Autodesk Fusion 360 part; units mm, degrees
(part 2 of 2)
sketch "Sketch1" plane through (0, 0, 0) normal (0, 0, 1) x (1, 0, 0)
  circle A0 centre (0, 0) radius 13.65
  circle A1 centre (0, 0) radius 18.65
  line L0 (0, 0) -> (0, 18.65)
  line L1 (0, 0) -> (0, -18.65)
  line L2 (-0.5, -18.6433) -> (-0.5, 18.6433)
  line L3 (-0.5, 18.6433) -> (-0.5, 25.4071)
  line L4 (-0.5, 25.4071) -> (-3, 25.4071)
  line L5 (-3, 25.4071) -> (-3, 18.4071)
  line L6 (0, 0) -> (-1.65, 0) construction
  line L7 (-1.65, 0) -> (-18.65, 0) construction
  line L8 (-18.216, 4) -> (-32, 4)
  line L9 (-32, 4) -> (-32, -4)
  line L10 (-32, -4) -> (-18.216, -4)
  circle A2 centre (-28, 0) radius 2.5
  circle A3 centre (-22, 0) radius 2.5
  line L11 (-22, -2.5) -> (-28, -2.5)
  line L12 (-28, 2.5) -> (-22, 2.5)
  line L13 (0.5, -18.6433) -> (0.5, 18.6433)
  line L14 (0.5, 18.6433) -> (0.5, 25.4071)
  line L15 (0.5, 25.4071) -> (3, 25.4071)
  line L16 (3, 25.4071) -> (3, 18.4071)
  line L17 (18.216, 4) -> (32, 4)
  circle A4 centre (22, 0) radius 2.5
  line L18 (28, 2.5) -> (22, 2.5)
  line L19 (22, -2.5) -> (28, -2.5)
  circle A5 centre (28, 0) radius 2.5
  line L20 (32, -4) -> (18.216, -4)
  line L21 (32, 4) -> (32, -4)
  dimension "d1" = 27.3
  dimension "d2" = 5
  dimension "d3" = 0.5
  dimension "d4" = 2.5
  dimension "d5" = 7
  dimension "d6" = 8
  dimension "d7" = 4
  dimension "d8" = 32
  dimension "d9" = 5
  dimension "d10" = 5
  dimension "d11" = 6
  dimension "d12" = 22
  constraint coincident A0.centre A1.centre
  constraint coincident A1 L0.end
  constraint vertical L0
  constraint coincident A1 L1.end
  constraint parallel L0 L1
  constraint coincident A1 L2.start
  constraint coincident A1 L2.end
  constraint parallel L1 L2
  constraint parallel L2 L3
  constraint perpendicular L3 L4
  constraint coincident A1 L5.end
  constraint perpendicular L4 L5
  constraint perpendicular L0 L6
  constraint coincident A1 L7.end
  constraint perpendicular L0 L7
  constraint coincident A1 L8.start
  constraint perpendicular L2 L8
  constraint perpendicular L8 L9
  constraint coincident A1 L10.end
  constraint perpendicular L9 L10
  constraint coincident A3 L11.start
  constraint coincident A2 L11.end
  constraint parallel L10 L11
  constraint coincident A2 L12.start
  constraint coincident A3 L12.end
  constraint parallel L11 L12
  constraint horizontal A0.centre A3.centre
  constraint horizontal A2.centre A3.centre
  constraint tangent A2 L12
  constraint tangent A3 L11
  constraint symmetric L0 L2.start L13.start
  constraint symmetric L0 L2.end L13.end
  constraint symmetric L0 L3.end L14.end
  constraint symmetric L0 L4.end L15.end
  constraint symmetric L0 L5.end L16.end
  constraint symmetric L0 L8.start L17.start
  constraint symmetric L0 L8.end L17.end
  constraint symmetric L0 L9.end L20.start
  constraint symmetric L0 L10.end L20.end
  constraint symmetric L0 A2 A5
  constraint symmetric L0 A3 A4
  constraint symmetric L0 L11.start L19.start
  constraint symmetric L0 L11.end L19.end
  constraint symmetric L0 L12.start L18.start
  constraint symmetric L0 L12.end L18.end
  measures "d1" diameter of A0
  measures "d2" distance of A0 A1
  measures "d3" distance of L0 L2
  measures "d4" distance of L3.end L4.end
  measures "d5" distance of L4.end L5.end
  measures "d6" distance of L8 L10
  measures "d7" distance of A0.centre L8
  measures "d8" distance of A0.centre L9
  measures "d9" diameter of A2
  measures "d10" diameter of A3
  measures "d11" distance of A2.centre A3.centre
  measures "d12" distance of A0.centre A3.centre
extrude "Extrude1" add sketch "Sketch1" along normal blind 5 contours A0 A1 L13 | A0 A1 L1 L13 | A1 L14 L15 L16 | A0 A1 L1 L2 | A0 A1 L2 | A1 L17 L20 L21 | A1 L3 L4 L5 | A1 L8 L9 L10
fillet "Fillet1" radius 4 1 edges at (-3, 18.4071, 2.5)
fillet "Fillet2" radius 3 4 edges at (-32, -4, 2.5) (-32, 4, 2.5) (-18.216, 4, 2.5) (-18.216, -4, 2.5)
fillet "Fillet3" radius 1 1 edges at (-0.5, 13.6408, 2.5)
fillet "Fillet4" radius 1 2 edges at (-1.75, 25.4071, 5) (-1.75, 25.4071, 0)
fillet "Fillet5" radius 3 4 edges at (18.216, -4, 2.5) (32, -4, 2.5) (32, 4, 2.5) (18.216, 4, 2.5)
fillet "Fillet6" radius 4 1 edges at (3, 18.4071, 2.5)
fillet "Fillet7" radius 1 2 edges at (1.75, 25.4071, 5) (1.75, 25.4071, 0)
fillet "Fillet8" radius 1 1 edges at (0.5, 13.6408, 2.5)
sketch "Sketch2" plane through (-0.5, 0, 0) normal (1, 0, 0) x (0, 1, 0)
  arc A0 (24.4071, 0) -> (25.4071, 1) centre (24.4071, 1) ccw
  line L0 (25.4071, 1) -> (25.4071, 4)
  arc A1 (25.4071, 4) -> (24.4071, 5) centre (24.4071, 4) ccw
  line L1 (24.4071, 5) -> (18.6433, 5)
  line L2 (18.6433, 5) -> (18.6433, 0)
  line L3 (18.6433, 0) -> (24.4071, 0)
  circle A2 centre (22.4071, 2.5) radius 1.5
  dimension "d23" = 3
  dimension "d24" = 3
  dimension "d25" = 2.5
  measures "d23" diameter of A2
  measures "d24" distance of L0 A2.centre
  measures "d25" distance of L1 A2.centre
extrude "Extrude2" cut sketch "Sketch2" along normal mid plane 10 contours A2

design "Pillar 45mm"
Autodesk Fusion 360 part; units mm, degrees
sketch "Sketch1" plane through (0, 0, 0) normal (0, 0, 1) x (1, 0, 0)
  line L0 (-1.4434, 2.5) -> (-2.8868, 0)
  line L1 (-2.8868, 0) -> (-1.4434, -2.5)
  line L2 (-1.4434, -2.5) -> (1.4434, -2.5)
  line L3 (1.4434, -2.5) -> (2.8868, 0)
  line L4 (2.8868, 0) -> (1.4434, 2.5)
  line L5 (1.4434, 2.5) -> (-1.4434, 2.5)
  dimension "d1" = 5
  measures "d1" distance of L0 L3
extrude "Extrude1" add sketch "Sketch1" along normal blind 45
sketch "Sketch2" plane through (0, 0, 45) normal (0, 0, 1) x (-1, 0, 0)
  line L0 (-1.4434, -2.5) -> (1.4434, -2.5)
  line L1 (1.4434, -2.5) -> (2.8868, 0)
  line L2 (2.8868, 0) -> (1.4434, 2.5)
  line L3 (1.4434, 2.5) -> (-1.4434, 2.5)
  line L4 (-1.4434, 2.5) -> (-2.8868, 0)
  line L5 (-2.8868, 0) -> (-1.4434, -2.5)
  circle A0 centre (0, 0) radius 1.5
  dimension "d4" = 3
  constraint coincident A0.centre origin
  measures "d4" diameter of A0
extrude "Extrude2" cut sketch "Sketch2" against normal blind 8 contours A0
sketch "Sketch3" plane through (0, 0, 0) normal (0, 0, -1) x (1, 0, 0)
  line L0 (-1.4434, -2.5) -> (1.4434, -2.5)
  line L1 (1.4434, -2.5) -> (2.8868, 0)
  line L2 (2.8868, 0) -> (1.4434, 2.5)
  line L3 (1.4434, 2.5) -> (-1.4434, 2.5)
  line L4 (-1.4434, 2.5) -> (-2.8868, 0)
  line L5 (-2.8868, 0) -> (-1.4434, -2.5)
  circle A0 centre (0, 0) radius 1.5
  dimension "d7" = 3
  constraint coincident A0.centre origin
  measures "d7" diameter of A0
extrude "Extrude3" cut sketch "Sketch3" against normal blind 8 contours A0
thread "Thread1" "ISO Metric profile 3.0 M3x0.5 M3x0.5 6H" major diameter 3.086 minor diameter 2.529 pitch 0.5 angle 60 resizes the face on face at (1.4981, 0.0748, 5.3333) on face at (-1.4925, 0.1494, 42.3333)
